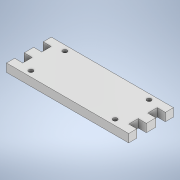
# Autodesk Inventor part: camMountBacking
Saved by Autodesk Inventor 2020 (Build 240168000, 168)
## iProperties
Created: 2019-08-05
Part Number: camMountBacking
Material: Generic
Document SubType Name: Modeling
Designer: n10208577
Density: 1 g/cm^3
Appearance: Default
Author: n10208577
Autodesk Inventor part; units mm, degrees
ref_plane "YZ Plane" through (0, 0, 0) normal (1, 0, 0) x (0, 1, 0)
ref_plane "XZ Plane" through (0, 0, 0) normal (0, 1, 0) x (-1, 0, 0)
ref_plane "XY Plane" through (0, 0, 0) normal (0, 0, 1) x (1, 0, 0)
sketch "Sketch1" plane through (0, 0, 0) normal (0, 1, 0) x (-1, 0, 0)
  circle A0 centre (-17.1731, 6.5813) radius 0.8
  circle A1 centre (-17.1731, -5.9187) radius 0.8
  circle A2 centre (13.8269, 6.5813) radius 0.8
  circle A3 centre (13.8269, -5.9187) radius 0.8
  line L0 (-21.1731, 5.5813) -> (-21.1731, 2.0813)
  line L1 (-21.1731, -1.4187) -> (-21.1731, -4.9187)
  line L2 (17.8269, 5.5813) -> (17.8269, 2.0813)
  line L3 (17.8269, -1.4187) -> (17.8269, -4.9187)
  line L4 (-24.1731, 8.5813) -> (20.8269, 8.5813)
  line L5 (20.8269, -7.9187) -> (-24.1731, -7.9187)
  line L6 (-24.1731, -7.9187) -> (-24.1731, -4.9187)
  line L7 (-24.1731, -4.9187) -> (-21.1731, -4.9187)
  line L8 (-24.1731, 8.5813) -> (-24.1731, 5.5813)
  line L9 (-24.1731, 5.5813) -> (-21.1731, 5.5813)
  line L10 (-24.1731, -1.4187) -> (-21.1731, -1.4187)
  line L11 (-24.1731, 2.0813) -> (-21.1731, 2.0813)
  line L12 (-24.1731, -1.4187) -> (-24.1731, 2.0813)
  line L13 (20.8269, -7.9187) -> (20.8269, -4.9187)
  line L14 (20.8269, -4.9187) -> (17.8269, -4.9187)
  line L15 (20.8269, 8.5813) -> (20.8269, 5.5813)
  line L16 (20.8269, 5.5813) -> (17.8269, 5.5813)
  line L17 (20.8269, -1.4187) -> (17.8269, -1.4187)
  line L18 (20.8269, 2.0813) -> (17.8269, 2.0813)
  line L19 (20.8269, -1.4187) -> (20.8269, 2.0813)
  point P0 (0, 0)
  constraints: 40 end point, 4 centre point
extrude "Extrusion1" add sketch "Sketch1" along normal blind 3
body "Solid1"
